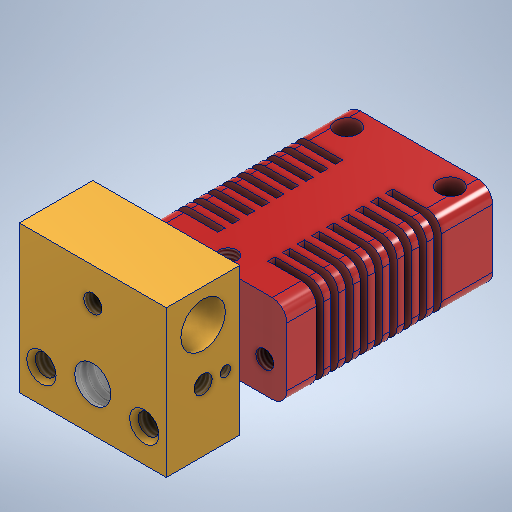
# Autodesk Inventor part: Hotend
Saved by Autodesk Inventor 2025 (Build 290162000, 162)
## iProperties
Created: 2025-01-29
Part Number: Hotend
Material: Aluminum 6061
Document SubType Name: Modeling
Designer: MAL16204
Density: 2.7 g/cm^3
Appearance: Aluminum - Flat
Mass: 19.9278 g
Surface Area: 80.2197 cm^2
Volume: 7.38065 cm^3
Author: MAL16204
Autodesk Inventor part; units mm, degrees
note: some values were not read from the file. Chosen so that the rebuilt part matches the saved one: direction of "bottomScrewHoles"; direction of "filamentThroughHole".
ref_plane "YZ Plane" through (0, 0, 0) normal (1, 0, 0) x (0, 1, 0)
sketch "Sketch6" plane through (0, 0, 0) normal (0, 1, 0) x (-1, 0, 0)
  line L0 (10, -14) -> (-10, -14)
  line L1 (-10, -14) -> (-10, 14)
  line L2 (-10, 14) -> (10, 14)
  line L3 (10, 14) -> (10, -14)
  line L4 (10, -14) -> (-10, 14) construction
  line L5 (-10, -14) -> (10, 14) construction
  point P0 (0, 0)
  dimension "d13" = 28
  dimension "d14" = 20
  constraints: 12 end point, 2 midpoint, 2 parallel, 1 horizontal, 1 perpendicular
  measures "d13" distance of L0.end L1.end
  measures "d14" distance of L1.end L2.end
extrude "mainBodyExtrude" add sketch "Sketch6" along normal blind 12
fillet "cornerFillets" radius 2 4 edges at (-10, 12, 0) (-10, 0, 0) (10, 12, 0) (10, 0, 0)
sketch "Sketch7" plane through (0, 12, 0) normal (0, 1, 0) x (1, 0, 0)
  line L0 (-10, 14) -> (-10, -14) projected
  line L1 (-10, 7) -> (-3.4, 7)
  line L2 (-3.4, 7) -> (-3.4, 6)
  line L3 (-3.4, 6) -> (-10, 6)
  line L4 (-10, 6) -> (-10, 7)
  line L5 (10, 14) -> (-10, 14) projected
  line L6 (10, 6) -> (3.4, 6)
  line L7 (3.4, 7) -> (10, 7)
  line L8 (10, 7) -> (10, 6)
  line L9 (3.4, 6) -> (3.4, 7)
  line L10 (-3.4, 4) -> (-10, 4)
  line L11 (-10, 5) -> (-3.4, 5)
  line L12 (-3.4, 5) -> (-3.4, 4)
  line L13 (-10, 4) -> (-10, 5)
  line L14 (10, 4) -> (3.4, 4)
  line L15 (3.4, 5) -> (10, 5)
  line L16 (10, 5) -> (10, 4)
  line L17 (3.4, 4) -> (3.4, 5)
  line L18 (-3.4, 2) -> (-10, 2)
  line L19 (-10, 3) -> (-3.4, 3)
  line L20 (-3.4, 3) -> (-3.4, 2)
  line L21 (-10, 2) -> (-10, 3)
  line L22 (10, 2) -> (3.4, 2)
  line L23 (3.4, 3) -> (10, 3)
  line L24 (10, 3) -> (10, 2)
  line L25 (3.4, 2) -> (3.4, 3)
  line L26 (-3.4, 0) -> (-10, 0)
  line L27 (-10, 1) -> (-3.4, 1)
  line L28 (-3.4, 1) -> (-3.4, 0)
  line L29 (-10, 0) -> (-10, 1)
  line L30 (10, 0) -> (3.4, 0)
  line L31 (3.4, 1) -> (10, 1)
  line L32 (10, 1) -> (10, 0)
  line L33 (3.4, 0) -> (3.4, 1)
  line L34 (-3.4, -2) -> (-10, -2)
  line L35 (-10, -1) -> (-3.4, -1)
  line L36 (-3.4, -1) -> (-3.4, -2)
  line L37 (-10, -2) -> (-10, -1)
  line L38 (10, -2) -> (3.4, -2)
  line L39 (3.4, -1) -> (10, -1)
  line L40 (10, -1) -> (10, -2)
  line L41 (3.4, -2) -> (3.4, -1)
  line L42 (-3.4, -4) -> (-10, -4)
  line L43 (-10, -3) -> (-3.4, -3)
  line L44 (-3.4, -3) -> (-3.4, -4)
  line L45 (-10, -4) -> (-10, -3)
  line L46 (10, -4) -> (3.4, -4)
  line L47 (3.4, -3) -> (10, -3)
  line L48 (10, -3) -> (10, -4)
  line L49 (3.4, -4) -> (3.4, -3)
  line L50 (-3.4, -6) -> (-10, -6)
  line L51 (-10, -5) -> (-3.4, -5)
  line L52 (-3.4, -5) -> (-3.4, -6)
  line L53 (-10, -6) -> (-10, -5)
  line L54 (10, -6) -> (3.4, -6)
  line L55 (3.4, -5) -> (10, -5)
  line L56 (10, -5) -> (10, -6)
  line L57 (3.4, -6) -> (3.4, -5)
  line L58 (-3.4, -8) -> (-10, -8)
  line L59 (-10, -7) -> (-3.4, -7)
  line L60 (-3.4, -7) -> (-3.4, -8)
  line L61 (-10, -8) -> (-10, -7)
  line L62 (10, -8) -> (3.4, -8)
  line L63 (3.4, -7) -> (10, -7)
  line L64 (10, -7) -> (10, -8)
  line L65 (3.4, -8) -> (3.4, -7)
  line L66 (-3.4, -10) -> (-10, -10)
  line L67 (-10, -9) -> (-3.4, -9)
  line L68 (-3.4, -9) -> (-3.4, -10)
  line L69 (-10, -10) -> (-10, -9)
  line L70 (10, -10) -> (3.4, -10)
  line L71 (3.4, -9) -> (10, -9)
  line L72 (10, -9) -> (10, -10)
  line L73 (3.4, -10) -> (3.4, -9)
  point P0 (0, 0)
  point P1 (-10, -6)
  point P2 (-10, -8)
  dimension "d17" = 1
  dimension "d18" = 6.6
  dimension "d19" = 7
  dimension "d22" = 13.4
  dimension "d25" = 2
  constraints: 144 end point, 64 vertical alignment, 34 parallel, 32 collinear, 2 horizontal, 1 perpendicular, 10 other
  measures "d17" distance of L1.end L2.end
  measures "d18" distance of L1.start L1.end
  measures "d19" distance between parallel lines of L5 L1
  measures "d22" distance of L2.end L6.start
  measures "d25" distance of L2.end L10.start
extrude "finsExtrude" cut sketch "Sketch7" against normal blind 12
sketch "Sketch8" plane through (0, 12, 0) normal (0, 1, 0) x (1, 0, 0)
  line L0 (0, 0) -> (0, 47.2841) construction
  line L1 (-7, 11.1844) -> (7, 11.1844) construction
  dimension "d31" = 14
  constraints: 4 end point, 1 horizontal, 1 horizontal alignment, 1 vertical
  measures "d31" distance of L1.end L1.start
hole "topHoles" at (7, 12, -11.1844) at (-7, 12, -11.1844) direction (0, -1, 0) diameter 3.2 end through all
sketch "Sketch9" plane through (0, 12, 0) normal (0, 1, 0) x (1, 0, 0)
  line L0 (0, 0) -> (0, -23.0152) construction
  line L1 (8, -10) -> (3.4, -10) construction
  line L2 (4.4061, -10) -> (4.4061, -14) construction
  line L3 (-8, -14) -> (8, -14) construction
  point P0 (0, -12)
  point P1 (4.4061, -12)
  constraints: 4 end point, 3 point on line, 2 vertical, 1 horizontal alignment, 1 midpoint
hole "bottomTensionScrewHole" at (0, 12, 12) direction (0, -1, 0) diameter 2.459 end through all thread size "M3x0.5" class "6H" standard "ISO Metric profile"
sketch "Sketch11" plane through (-8, 0, 14) normal (0, 0, 1) x (1, 0, 0)
  line L0 (-2, 2) -> (-2, 10) construction
  line L1 (18, 2) -> (18, 10) construction
  line L2 (0, 12) -> (16, 12) construction
  line L3 (-2, 6) -> (8, 6) construction
  line L4 (1, 6) -> (1, 0) construction
  line L5 (4.6, 0) -> (0, 0) construction
  line L6 (15, 6) -> (15, 1.7949) construction
  line L7 (1, 4.239) -> (15, 4.239) construction
  point P0 (8, 0)
  dimension "d54" = 14
  constraints: 8 end point, 4 point on line, 3 coincident, 2 parallel, 2 vertical, 1 midpoint, 1 perpendicular, 1 other
  measures "d54" distance between parallel lines of L6 L4
hole "bottomScrewHoles" at (-7, 4.239, 14) at (7, 4.239, 14) direction (0, 0, -1) diameter 2.459 depth 4 thread size "M3x0.5" class "6H" standard "ISO Metric profile"
hole "filamentThroughHole" at (0, 6, 14) direction (0, 0, -1) diameter 6.8 depth 28
ref_plane "Work Plane1" through (8, 0, 0.4) normal (0, 0, -1) x (-1, 0, 0)
sketch "Sketch12" plane through (8, 0, 0.4) normal (0, 0, -1) x (-1, 0, 0)
  circle A0 centre (8, 6) radius 2.15
  line L0 (11.4, 6) -> (11.4, 0) projected
  circle A1 centre (8, 6) radius 3.4
  point P0 (8, 0)
  dimension "d70" = 4.3
  constraints: 1 centre point, 1 coincident, 1 horizontal alignment, 2 other
  measures "d70" diameter of A0
extrude "insideFilamentChannelExtrude" add sketch "Sketch12" against normal blind 25
ref_plane "Work Plane2" through (0, 6, 20.4) normal (0, 0, 1) x (1, 0, 0)
sketch "Sketch13" plane through (0, 6, 20.4) normal (0, 0, 1) x (1, 0, 0)
  line L0 (10, 14) -> (-10, 14)
  line L1 (-10, 14) -> (-10, -6)
  line L2 (-10, -6) -> (10, -6)
  line L3 (10, -6) -> (10, 14)
  line L4 (10, 0) -> (-10, 0) construction
  line L5 (0, 14) -> (0, -6) construction
  point P0 (0, 0)
  point P1 (7, -1.5)
  point P2 (-7, -1.5)
  point P3 (0, 0)
  point P4 (0, 0)
  point P5 (0, 0)
  dimension "d93" = 20
  dimension "d94" = 20
  dimension "d95" = 6
  constraints: 12 end point, 3 coincident, 3 midpoint, 3 point on line, 2 parallel, 2 perpendicular, 1 horizontal, 1 horizontal alignment, 1 other
  measures "d93" distance of L0.start L0.end
  measures "d94" distance of L2.end L0.start
  measures "d95" distance between parallel lines of L2 L4
extrude "heaterBlockExtrude" add sketch "Sketch13" along normal blind 10
sketch "Sketch15" plane through (10, 0, 20.4) normal (1, 0, 0) x (0, 0, -1)
  line L0 (0, 0) -> (-10, 0) construction
  line L1 (-5, 0) -> (-5, 20) construction
  line L2 (0, 20) -> (-10, 20) construction
  circle A0 centre (-5, 15.5) radius 3.025
  line L3 (0, 0) -> (0, 20) construction
  line L4 (0, 8.5) -> (-10, 8.5) construction
  line L5 (-10, 20) -> (-10, 0) construction
  point P0 (20.4, 0)
  point P1 (-1.975, 8.5)
  dimension "d103" = 6.05
  dimension "d105" = 4.5
  dimension "d117" = 11.5
  constraints: 4 end point, 4 point on line, 2 midpoint, 1 centre point, 1 horizontal
  measures "d103" diameter of A0
  measures "d105" distance from line of L2 A0.centre
  measures "d117" distance between parallel lines of L4 L2
extrude "heaterElementHole" cut sketch "Sketch15" against normal through all
sketch "Sketch16" plane through (10, 0, 20.4) normal (1, 0, 0) x (0, 0, -1)
  line L0 (0, 20) -> (-10, 20) projected
  line L1 (-10, 0) -> (-10, 20) projected
  point P0 (20.4, 0)
  point P1 (-5, 8.5)
  dimension "d108" = 11.5
  dimension "d109" = 5
  measures "d108" distance from line of L0 point (-5, 8.5)
  measures "d109" distance from line of L1 point (-5, 8.5)
hole "retentionScrewHole" at (10, 8.5, 25.4) direction (-1, 0, 0) diameter 2.459 depth 15 thread size "M3x0.5" class "6H" standard "ANSI Metric M Profile"
hole "thermoresistorHole" at (10, 8.5, 22.375) direction (-1, 0, 0) diameter 1.4211 depth 5.7 tip angle 118 thread size "M1.8x0.35" class "6H" standard "ANSI Metric M Profile"
sketch "Sketch17" plane through (0, 6, 30.4) normal (0, 0, 1) x (1, 0, 0)
  line L0 (10, 14) -> (-10, 14) construction
  line L1 (0, 14) -> (0, -6) construction
  line L2 (10, 9.5) -> (-10, 9.5) construction
  line L3 (-10, 14) -> (-10, -6) construction
  line L4 (-10, -6) -> (10, -6) construction
  line L5 (7, -1.5) -> (-7, -1.5) construction
  line L6 (-7, -1.5) -> (-10, -1.5) construction
  line L7 (7, -1.5) -> (10, -1.5) construction
  line L8 (10, -6) -> (10, 14) construction
  line L9 (10, 0) -> (-10, 0) construction
  point P0 (0, 9.5)
  point P1 (0, 0)
  dimension "d125" = 15.5
  dimension "d126" = 14
  dimension "d127" = 4.5
  dimension "d128" = 6
  constraints: 13 end point, 7 point on line, 3 midpoint, 2 horizontal, 2 perpendicular, 1 coincident, 1 collinear, 1 vertical
  measures "d125" distance between parallel lines of L4 L2
  measures "d126" distance of L5.start L5.end
  measures "d127" distance between parallel lines of L4 L5
  measures "d128" distance between parallel lines of L4 L9
hole "heaterElementRetentionScrew" at (0, 15.5, 30.4) direction (0, 0, -1) diameter 2.459 depth 4.05 thread size "M3x0.5" class "6H" standard "ANSI Metric M Profile"
hole "antispinScrewHoles" at (7, 4.5, 30.4) at (-7, 4.5, 30.4) direction (0, 0, -1) diameter 2.85 depth 10.4 countersink diameter 4 countersink angle 90 thread size "M3.5x0.6" class "6H" standard "ANSI Metric M Profile"
hole "nozzleHole" at (0, 6, 30.4) direction (0, 0, -1) diameter 4.917 depth 17.1 thread size "M6x1" class "6H" standard "ANSI Metric M Profile"
